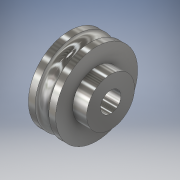
# Autodesk Inventor part: 1.5in pulley roller
Saved by Autodesk Inventor 2017 (Build 210142000, 142)
## iProperties
Created: 2017-01-17
Part Number: 1.5in pulley roller
Material: Generic
Document SubType Name: Modeling
Designer: Ben
Density: 1 g/cm^3
Appearance: Chrome - Polished
Author: Ben
Autodesk Inventor part; units mm, degrees
ref_plane "YZ Plane" through (0, 0, 0) normal (1, 0, 0) x (0, 1, 0)
ref_plane "XZ Plane" through (0, 0, 0) normal (0, 1, 0) x (-1, 0, 0)
ref_plane "XY Plane" through (0, 0, 0) normal (0, 0, 1) x (1, 0, 0)
sketch "Sketch1" plane through (0, 0, 0) normal (0, 0, 1) x (1, 0, 0)
  arc A0 (-3.175, 19.05) -> (3.175, 19.05) centre (0, 19.05) ccw
  line L0 (-3.175, 19.05) -> (-6.35, 19.05)
  line L1 (-6.35, 19.05) -> (-6.35, 4.7625)
  line L2 (3.175, 19.05) -> (6.35, 19.05)
  line L3 (0, 19.05) -> (0, 0) construction
  line L4 (-6.35, 4.7625) -> (12.8524, 4.7625)
  line L5 (12.8524, 4.7625) -> (12.8524, 11.1125)
  line L6 (12.8524, 11.1125) -> (6.35, 11.1125)
  line L7 (6.35, 11.1125) -> (6.35, 19.05)
  line L8 (0, 0) -> (15.9105, 0) construction
  dimension "d2" = 3.175
  dimension "d3" = 3.175
  dimension "d4" = 4.7625
  dimension "d5" = 6.5024
  dimension "d6" = 6.35
  dimension "d7" = 19.05
  constraints: 18 end point, 4 perpendicular, 3 horizontal, 2 line through centre, 2 point on circle, 1 centre point, 1 collinear, 1 point on line, 1 vertical
  measures "d2" radius of A0
  measures "d3" distance of L0.start L0.end
  measures "d4" distance from line of L3.end L4
  measures "d5" distance of L5.end L6.end
  measures "d6" distance between parallel lines of L4 L6
  measures "d7" distance of L3.start L3.end
revolve "Revolution1" add sketch "Sketch1" angle 360 about axis through (0, 0, 0) along (1, 0, 0)
body "Solid1"
